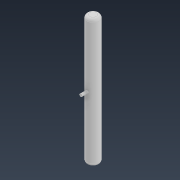
# Autodesk Inventor part: Part2pasador
Saved by Autodesk Inventor 2021.2 (Build 252289000, 289)
## iProperties
Created: 2026-09-01
Part Number: Part2pasador
Material: Generic
Document SubType Name: Modeling
Designer: Tecnica
Density: 1 g/cm^3
Appearance: Default
Author: Tecnica
Autodesk Inventor part; units mm, degrees
ref_plane "YZ Plane" through (0, 0, 0) normal (1, 0, 0) x (0, 1, 0)
ref_plane "XZ Plane" through (0, 0, 0) normal (0, 1, 0) x (-1, 0, 0)
ref_plane "XY Plane" through (0, 0, 0) normal (0, 0, 1) x (1, 0, 0)
sketch "Sketch1" plane through (0, 0, 0) normal (0, 1, 0) x (-1, 0, 0)
  circle A0 centre (0, 0) radius 4.5
  dimension "d0" = 9
  constraints: 1 centre point, 1 coincident
  measures "d0" diameter of A0
extrude "Extrusion1" add sketch "Sketch1" along normal mid plane 95
fillet "Fillet1" radius 2 2 edges at (4.5, 47.5, 0) (4.5, -47.5, 0)
sketch "Sketch2" plane through (0, 0, 0) normal (0, 0, 1) x (1, 0, 0)
  circle A0 centre (0, 0) radius 1
  dimension "d4" = 2
  constraints: 1 centre point, 1 coincident
  measures "d4" diameter of A0
extrude "Extrusion2" add sketch "Sketch2" along normal blind 9 and the other way blind 4.5
body "Solid1"
